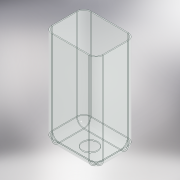
# Autodesk Inventor part: silo
Saved by Autodesk Inventor 2020 (Build 240168000, 168)
## iProperties
Created: 2020-06-18
Part Number: silo
Material: Generic
Document SubType Name: Modeling
Designer: pc-konvi
Density: 1 g/cm^3
Appearance: Clear
Author: pc-konvi
Autodesk Inventor part; units mm, degrees
ref_plane "YZ Plane" through (0, 0, 0) normal (1, 0, 0) x (0, 1, 0)
ref_plane "XZ Plane" through (0, 0, 0) normal (0, 1, 0) x (-1, 0, 0)
ref_plane "XY Plane" through (0, 0, 0) normal (0, 0, 1) x (1, 0, 0)
sketch "Sketch1" plane through (0, 0, 0) normal (0, 0, 1) x (1, 0, 0)
  line L0 (52.5, 200) -> (-52.5, 200)
  line L1 (-52.5, 200) -> (-52.5, 0)
  line L2 (-52.5, 0) -> (52.5, 0)
  line L3 (52.5, 0) -> (52.5, 200)
  point P0 (0, 0)
  point P1 (0, 0)
  dimension "d0" = 105
  dimension "d1" = 200
  constraints: 8 end point, 2 coincident, 2 parallel, 1 horizontal, 1 midpoint, 1 perpendicular
  measures "d0" distance of L1.end L2.end
  measures "d1" distance of L2.end L0.start
extrude "Extrusion1" add sketch "Sketch1" along normal mid plane 80
fillet "Fillet1" radius 15 8 edges at (52.5, 100, 40) (52.5, 100, -40) (-52.5, 100, 40) (-52.5, 100, -40) (0, 0, 40) (-52.5, 0, 0) (0, 0, -40) (52.5, 0, 0)
shell "Shell1" thickness 2 removed faces 1 at (-12.5, 200, 13.3333)
sketch "Sketch2" plane through (-37.5, 0, 25) normal (0, -1, 0) x (1, 0, 0)
  circle A0 centre (37.5, -25) radius 17.3802 construction
  circle A1 centre (37.5, -25) radius 15.3802
  dimension "d6" = 2
  constraints: 2 centre point, 1 coincident
  measures "d6" radial gap between concentric circles of A0 A1
extrude "Extrusion2" cut sketch "Sketch2" against normal blind 5
body "Solid1"
